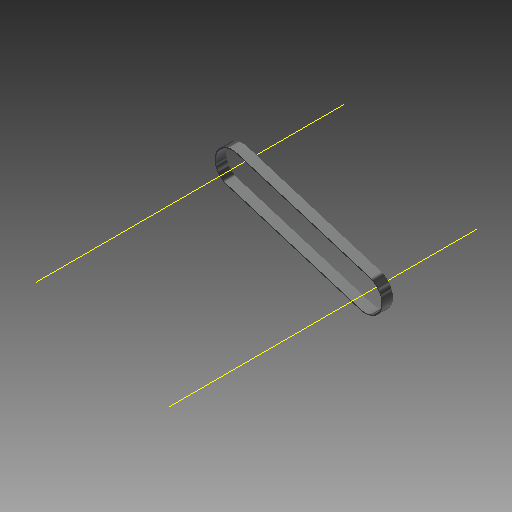
# Autodesk Inventor part: Zahnriemen
Saved by Autodesk Inventor 2017.3 (Build 213256000, 256)
## iProperties
Created: 2018-02-01
Part Number: Zahnriemen
Material: Rubber
Document SubType Name: Modeling
Designer: Dima
Density: 1 g/cm^3
Appearance: Rubber - Black - Version 1.1
CustomPartVersion: 1
Author: Dima
Autodesk Inventor part; units mm, degrees
sketch "Skizzenpfad" plane through (0, 0, 0) normal (0, 0, 1) x (1, 0, 0)
  arc A0 (1.6451, -22.8731) -> (11.0463, 7.5379) centre (6.3457, -7.6676) ccw
  arc A1 (-115.2361, 46.5766) -> (-124.6373, 16.1656) centre (-119.9367, 31.3711) ccw
  line L0 (-115.2361, 46.5766) -> (11.0463, 7.5379)
  line L1 (1.6451, -22.8731) -> (-124.6373, 16.1656)
  constraints: 4 end point, 4 point on circle, 2 centre point
ref_plane "Querschnittsebene" through (11.0463, 7.5379, 0) normal (-0.9554, 0.2953, 0) x (0, 0, 1)
ref_plane "Arbeitsebene2" through (6.3457, -7.6676, 0) normal (-1, 0, 0) x (0, 0, 1)
ref_plane "Arbeitsebene3" through (-119.9367, 31.3711, 0) normal (0.8817, -0.4719, 0) x (0, 0, 1)
sketch "Querschnitt" plane through (11.0463, 7.5379, 0) normal (-0.9554, 0.2953, 0) x (0, 0, 1)
  line L0 (-5, 0.5) -> (5, 0.5)
  line L1 (5, 0.5) -> (5, -0.5)
  line L2 (5, -0.5) -> (-5, -0.5)
  line L3 (-5, -0.5) -> (-5, 0.5)
  line L4 (-5, 0) -> (5, 0) construction
  point P0 (0, 0)
  point P1 (0, 0)
  dimension "d0" = 10
  dimension "d4" = 0.5
  dimension "d5" = 0.5
  constraints: 10 end point, 3 midpoint, 2 parallel, 1 coincident, 1 horizontal, 1 perpendicular, 1 other
  measures "d0" distance between parallel lines of L1 L3
  measures "d4" distance between parallel lines of L2 L4
  measures "d5" distance between parallel lines of L4 L0
sweep "Riemen" add profiles "Querschnitt" path "Skizzenpfad"
equation "\"d0\" = da_B"
equation "\"d4\" = da_a"
equation "\"d5\" = da_a2"
equation "\"da_B\" = 10"
equation "\"da_pb\" = 5"
equation "\"da_L\" = 364.35771"
equation "\"da_a\" = 0.5"
equation "\"da_S\" = 2.65"
equation "\"da_Beta\" = 20deg"
equation "\"da_Ht\" = 1.2"
equation "\"da_H\" = 2.2"
equation "\"da_a2\" = 0.5"
body "Solid1"
